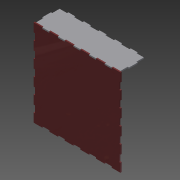
# Autodesk Inventor part: wordClock
Saved by Autodesk Inventor 2015 (Build 190159000, 159)
## iProperties
Created: 2015-02-10
Part Number: wordClock
Material: Generic
Document SubType Name: Modeling
Designer: Iain
Density: 1 g/cm^3
Appearance: Default
Author: Iain
Autodesk Inventor part; units mm, degrees
ref_plane "YZ Plane" through (0, 0, 0) normal (1, 0, 0) x (0, 1, 0)
ref_plane "XZ Plane" through (0, 0, 0) normal (0, 1, 0) x (-1, 0, 0)
ref_plane "XY Plane" through (0, 0, 0) normal (0, 0, 1) x (1, 0, 0)
sketch "Sketch1" plane through (0, 0, 0) normal (0, 0, 1) x (1, 0, 0)
  line L0 (-97, 97) -> (97, 97)
  line L1 (97, 97) -> (97, -97)
  line L2 (97, -97) -> (-97, -97)
  line L3 (-97, -97) -> (-97, 97)
  point P0 (0, 0)
  point P1 (0, 97)
  point P2 (-97, 0)
  dimension "FrontFaceWidth" = 194
  dimension "FrontFaceHeight" = 194
  constraints: 8 end point, 2 midpoint, 2 parallel, 1 horizontal, 1 horizontal alignment, 1 perpendicular, 1 vertical alignment
  measures "FrontFaceWidth" distance of L0.start L0.end
  measures "FrontFaceHeight" distance of L2.end L0.start
extrude "FrontFaceBase" add sketch "Sketch1" along normal mid plane 3
sketch "Sketch4" plane through (0, 0, 1.5) normal (0, 0, 1) x (1, 0, 0)
  line L0 (-100, 100) -> (-80, 100)
  line L1 (-80, 100) -> (-80, 97)
  line L2 (-80, 97) -> (-100, 97)
  line L3 (-100, 97) -> (-100, 100)
  point P0 (-97, 97)
  point P1 (0, 0)
  point P2 (-90, 97)
  dimension "d6" = 3
  dimension "FrontFaceTabWidth" = 20
  dimension "d8" = 3
  constraints: 8 end point, 2 parallel, 1 horizontal, 1 horizontal alignment, 1 midpoint, 1 perpendicular
  measures "d6" distance of point (-97, 97) L2.end
  measures "FrontFaceTabWidth" distance of L0.end L0.start
  measures "d8" distance of L1.end L0.end
extrude "Extrusion2" add sketch "Sketch4" against normal blind 3
pattern_linear "FrontTopTabs" count 6 spacing 36 along (1, 0, 0) of "Extrusion2"
sketch "Sketch5" plane through (0, 0, 1.5) normal (0, 0, 1) x (1, 0, 0)
  line L0 (-100, -100) -> (-97, -100)
  line L1 (-97, -100) -> (-97, -80)
  line L2 (-97, -80) -> (-100, -80)
  line L3 (-100, -80) -> (-100, -100)
  point P0 (-97, -97)
  point P1 (0, 0)
  point P2 (-97, -90)
  dimension "d14" = 3
  dimension "d15" = 3
  dimension "d16" = 20
  constraints: 8 end point, 2 parallel, 1 horizontal, 1 midpoint, 1 perpendicular, 1 vertical alignment
  measures "d14" distance of point (-97, -97) L0.end
  measures "d15" distance of L0.start L0.end
  measures "d16" distance of L2.end L0.start
extrude "Extrusion3" add sketch "Sketch5" against normal blind 3
pattern_linear "FontLeftTabs" count 6 spacing 36 along (0, 1, 0) of "Extrusion3"
mirror "FrontBottomTabs" about plane through (0, 0, 0) normal (0, 1, 0) of "Extrusion2", "FrontTopTabs"
mirror "FontRightTabs" about plane through (0, 0, 0) normal (1, 0, 0) of "Extrusion3", "FontLeftTabs"
sketch "Sketch6" plane through (-8, 97, -1.5) normal (0, 1, 0) x (1, 0, 0)
  line L0 (-92, -3) -> (108, -3)
  line L1 (108, -3) -> (108, 57)
  line L2 (108, 57) -> (-92, 57)
  line L3 (-92, 57) -> (-92, -3)
  point P0 (108, 27)
  dimension "TopFaceDepth" = 60
  constraints: 8 end point, 2 parallel, 1 coincident, 1 horizontal, 1 midpoint, 1 perpendicular, 1 vertical alignment
  measures "TopFaceDepth" distance of point (-92, -3) L2.end
extrude "TopFaceBase" add sketch "Sketch6" along normal blind 3 separate body
sketch "Sketch7" plane through (-8, 100, -1.5) normal (0, 1, 0) x (1, 0, 0)
  line L0 (-92, -3) -> (108, -3) projected
  line L1 (-92, 57) -> (-92, -3) projected
  line L2 (-92, -3) -> (-72, -3)
  line L3 (-72, -3) -> (-72, 0)
  line L4 (-72, 0) -> (-92, 0)
  line L5 (-92, 0) -> (-92, -3)
  point P0 (8, -1.5)
  point P1 (-92, 27)
  point P2 (8, -3)
  dimension "d25" = 20
  dimension "TopFaceFrontSlotDepth" = 3
  constraints: 8 end point, 2 midpoint, 2 parallel, 1 horizontal, 1 horizontal alignment, 1 perpendicular, 1 vertical alignment
  measures "d25" distance of L3.end L4.end
  measures "TopFaceFrontSlotDepth" distance of L2.start L4.end
extrude "Extrusion5" cut sketch "Sketch7" against normal blind 3 bodies 2
sketch "Sketch8" plane through (-8, 100, -1.5) normal (0, 1, 0) x (1, 0, 0)
  line L0 (108, -3) -> (105, -3)
  line L1 (105, -3) -> (105, 17)
  line L2 (105, 17) -> (108, 17)
  line L3 (108, 17) -> (108, -3)
  point P0 (8, -1.5)
  dimension "TopSideSlotWidth" = 20
  dimension "d33" = 3
  constraints: 8 end point, 2 parallel, 1 horizontal, 1 perpendicular
  measures "TopSideSlotWidth" distance of L0.end L1.end
  measures "d33" distance of L0.start L0.end
extrude "Extrusion6" cut sketch "Sketch8" against normal blind 3 bodies 2
pattern_linear "TopFrontSlots" count 6 spacing 36 along (1, 0, 0) of "Extrusion5", "Extrusion2" bodies 2
pattern_linear "TopSideRightSlots" count 2 spacing 40 along (0, 0, -1) of "Extrusion6" bodies 2
ref_plane "Work Plane1" through (-44, 100, -28.5) normal (0, 0, 1) x (1, 0, 0)
mirror "TopBackSlots" about plane through (-44, 100, -28.5) normal (0, 0, 1) of "Extrusion5", "Extrusion2", "TopFrontSlots" bodies 2
ref_plane "Work Plane2" through (0, 97, -18.5) normal (1, 0, 0) x (0, 0, -1)
mirror "TopSideLeftSlots" about plane through (0, 97, -18.5) normal (1, 0, 0) of "Extrusion6", "TopSideRightSlots" bodies 2
equation "\"FrontFaceWidth\" = ClockWidth - 2 * FrontFaceTabDepth"
equation "\"FrontFaceHeight\" = ClockHeight - 2 * FrontFaceTabDepth"
equation "\"FrontFaceThickness\" = Ply3mm"
equation "\"d6\" = TabDepth"
equation "\"FrontFaceTabWidth\" = TabWidth"
equation "\"d8\" = FrontFaceTabDepth"
equation "\"d9\" = FrontFaceThickness"
equation "\"d14\" = FrontFaceTabDepth"
equation "\"d15\" = FrontFaceTabDepth"
equation "\"d16\" = FrontFaceTabWidth"
equation "\"d17\" = FrontFaceThickness"
equation "\"TopFaceDepth\" = ClockDepth"
equation "\"TopFaceThickness\" = Ply3mm"
equation "\"d25\" = FrontFaceTabWidth"
equation "\"TopFaceFrontSlotDepth\" = FrontFaceThickness"
equation "\"d27\" = TopFaceThickness"
equation "\"d33\" = TabDepth"
equation "\"d34\" = TopFaceThickness"
equation "\"d38\" = FrontFaceTopTabSpacing"
equation "\"FrontFaceTabDepth\" = TabDepth"
equation "\"ClockDepth\" = 60"
equation "\"Ply3mm\" = 3"
equation "\"TabDepth\" = Ply3mm"
equation "\"TabWidth\" = 20"
equation "\"ClockWidth\" = 200"
equation "\"ClockHeight\" = 200"
equation "\"FrontFaceTopTabSpacing\" = 36"
body "Solid2"
